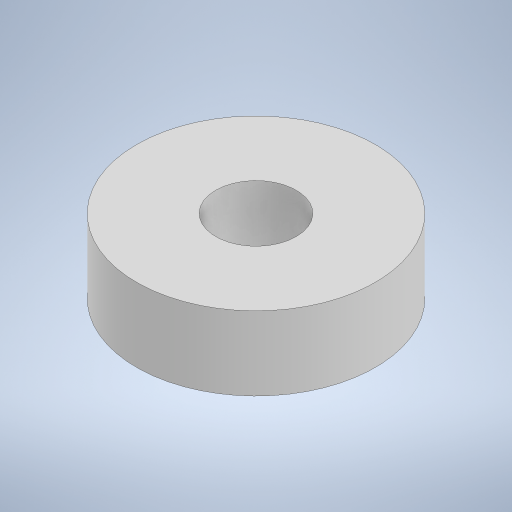
# Autodesk Inventor part: small bearing
Saved by Autodesk Inventor 2023 (Build 270158030, 158C)
## iProperties
Created: 2022-10-08
Part Number: small bearing
Material: Generic
Document SubType Name: Modeling
Designer: rm0990889
Density: 1 g/cm^3
Appearance: Default
Author: rm0990889
Autodesk Inventor part; units mm, degrees
ref_plane "YZ Plane" through (0, 0, 0) normal (1, 0, 0) x (0, 1, 0)
ref_plane "XZ Plane" through (0, 0, 0) normal (0, 1, 0) x (-1, 0, 0)
ref_plane "XY Plane" through (0, 0, 0) normal (0, 0, 1) x (1, 0, 0)
sketch "Sketch1" plane through (0, 0, 0) normal (0, 1, 0) x (-1, 0, 0)
  circle A0 centre (0, 0) radius 11.303
  circle A1 centre (0, 0) radius 3.81
  dimension "d0" = 22.606
  dimension "d1" = 7.62
  constraints: 2 centre point, 2 coincident
  measures "d0" diameter of A0
  measures "d1" diameter of A1
extrude "Extrusion1" add sketch "Sketch1" along normal blind 6.985
body "Solid1"
